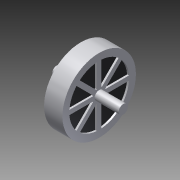
# Autodesk Inventor part: Wheel
Saved by Autodesk Inventor 2015 (Build 190159000, 159)
## iProperties
Created: 2015-01-08
Part Number: Wheel
Material: Generic
Document SubType Name: Modeling
Designer: Chandler Willoughby
Density: 1 g/cm^3
Appearance: Default
Author: Chandler Willoughby
Autodesk Inventor part; units mm, degrees
ref_plane "YZ Plane" through (0, 0, 0) normal (1, 0, 0) x (0, 1, 0)
ref_plane "XZ Plane" through (0, 0, 0) normal (0, 1, 0) x (-1, 0, 0)
ref_plane "XY Plane" through (0, 0, 0) normal (0, 0, 1) x (1, 0, 0)
sketch "Sketch1" plane through (0, 0, 0) normal (1, 0, 0) x (0, 1, 0)
  circle A0 centre (0, 0) radius 50.8
  dimension "d0" = 101.6
  constraints: 1 centre point, 1 coincident
  measures "d0" diameter of A0
extrude "Extrusion1" add sketch "Sketch1" along normal blind 25.4
sketch "Sketch2" plane through (25.4, 0, 0) normal (1, 0, 0) x (0, 0, -1)
  circle A0 centre (0, 0) radius 6.35
  dimension "d4" = 12.7
  constraints: 1 centre point, 1 coincident
  measures "d4" diameter of A0
extrude "Extrusion2" add sketch "Sketch2" along normal blind 33.3375
sketch "Sketch3" plane through (0, 0, 0) normal (-1, 0, 0) x (0, 0, 1)
  circle A0 centre (0, 0) radius 6.35
  constraints: 1 centre point, 1 coincident
extrude "Extrusion3" add sketch "Sketch3" along normal blind 33.3375
sketch "Sketch5" plane through (25.4, 0, 0) normal (1, 0, 0) x (0, 0, -1)
  circle A0 centre (0, 0) radius 44.45
  arc A1 (31.3429, -26.8561) -> (41.1529, -3.1727) centre (0, 0) ccw
  line L0 (0, 0) -> (82.55, 0) construction
  line L1 (41.1529, -3.1727) -> (8.9811, -3.1727)
  line L2 (31.3429, -26.8561) -> (82.1429, -26.8561) construction
  line L3 (31.3429, -26.8561) -> (8.594, -4.1072)
  line L4 (-4.1072, 8.594) -> (-4.5781, 9.0649)
  arc A2 (8.9811, -3.1727) -> (8.594, -4.1072) centre (8.9811, -3.7201) ccw
  arc A3 (41.1529, 3.1727) -> (31.3429, 26.8561) centre (0, 0) ccw
  line L5 (31.3429, 26.8561) -> (8.594, 4.1072)
  line L6 (41.1529, 3.1727) -> (8.9811, 3.1727)
  arc A4 (8.594, 4.1072) -> (8.9811, 3.1727) centre (8.9811, 3.7201) ccw
  arc A5 (26.8561, 31.3429) -> (3.1727, 41.1529) centre (0, 0) ccw
  line L7 (3.1727, 41.1529) -> (3.1727, 8.9811)
  line L8 (26.8561, 31.3429) -> (4.1072, 8.594)
  arc A6 (3.1727, 8.9811) -> (4.1072, 8.594) centre (3.7201, 8.9811) ccw
  arc A7 (-3.1727, 41.1529) -> (-26.8561, 31.3429) centre (0, 0) ccw
  line L9 (-26.8561, 31.3429) -> (-4.1072, 8.594)
  line L10 (-3.1727, 41.1529) -> (-3.1727, 8.9811)
  arc A8 (-4.1072, 8.594) -> (-3.1727, 8.9811) centre (-3.7201, 8.9811) ccw
  arc A9 (-31.3429, 26.8561) -> (-41.1529, 3.1727) centre (0, 0) ccw
  line L11 (-41.1529, 3.1727) -> (-8.9811, 3.1727)
  line L12 (-31.3429, 26.8561) -> (-8.594, 4.1072)
  arc A10 (-8.9811, 3.1727) -> (-8.594, 4.1072) centre (-8.9811, 3.7201) ccw
  arc A11 (-41.1529, -3.1727) -> (-31.3429, -26.8561) centre (0, 0) ccw
  line L13 (-31.3429, -26.8561) -> (-8.594, -4.1072)
  line L14 (-41.1529, -3.1727) -> (-8.9811, -3.1727)
  arc A12 (-8.594, -4.1072) -> (-8.9811, -3.1727) centre (-8.9811, -3.7201) ccw
  arc A13 (-26.8561, -31.3429) -> (-3.1727, -41.1529) centre (0, 0) ccw
  line L15 (-3.1727, -41.1529) -> (-3.1727, -8.9811)
  line L16 (-26.8561, -31.3429) -> (-4.1072, -8.594)
  arc A14 (-3.1727, -8.9811) -> (-4.1072, -8.594) centre (-3.7201, -8.9811) ccw
  arc A15 (3.1727, -41.1529) -> (26.8561, -31.3429) centre (0, 0) ccw
  line L17 (26.8561, -31.3429) -> (4.1072, -8.594)
  line L18 (3.1727, -41.1529) -> (3.1727, -8.9811)
  arc A16 (4.1072, -8.594) -> (3.1727, -8.9811) centre (3.7201, -8.9811) ccw
  dimension "d12" = 88.9
  dimension "d13" = 82.55
  dimension "d24" = 360
  constraints: 38 end point, 32 point on circle, 18 coincident, 17 centre point, 3 horizontal, 1 tangent, 95 other
  measures "d12" diameter of A0
  measures "d13" diameter of A1
extrude "Extrusion5" cut sketch "Sketch5" against normal blind 2.54 contours L3 A2 L1 A1 | L4 L9 A7 L10 A8 | L6 A4 L5 A3 | L8 A6 L7 A5 | L12 A10 L11 A9 | L14 A12 L13 A11 | L16 A14 L15 A13 | L18 A16 L17 A15
sketch "Sketch6" plane through (0, 0, 0) normal (-1, 0, 0) x (0, 0, 1)
  circle A0 centre (0, 0) radius 44.45
  arc A1 (-31.3429, 26.8561) -> (-41.1529, 3.1727) centre (0, 0) ccw
  line L0 (-8.594, 4.1072) -> (-31.3429, 26.8561) projected
  line L1 (-41.1529, 3.1727) -> (-8.9811, 3.1727)
  line L2 (-41.1529, 3.1727) -> (-8.9811, 3.1727) projected
  line L3 (-8.594, 4.1072) -> (-31.3429, 26.8561)
  arc A2 (-8.9811, 3.1727) -> (-8.594, 4.1072) centre (-8.9811, 3.7201) ccw
  arc A3 (-41.1529, -3.1727) -> (-31.3429, -26.8561) centre (0, 0) ccw
  line L4 (-31.3429, -26.8561) -> (-8.594, -4.1072)
  line L5 (-8.9811, -3.1727) -> (-41.1529, -3.1727)
  arc A4 (-8.594, -4.1072) -> (-8.9811, -3.1727) centre (-8.9811, -3.7201) ccw
  arc A5 (-26.8561, -31.3429) -> (-3.1727, -41.1529) centre (0, 0) ccw
  line L6 (-3.1727, -41.1529) -> (-3.1727, -8.9811)
  line L7 (-4.1072, -8.594) -> (-26.8561, -31.3429)
  arc A6 (-3.1727, -8.9811) -> (-4.1072, -8.594) centre (-3.7201, -8.9811) ccw
  arc A7 (3.1727, -41.1529) -> (26.8561, -31.3429) centre (0, 0) ccw
  line L8 (26.8561, -31.3429) -> (4.1072, -8.594)
  line L9 (3.1727, -8.9811) -> (3.1727, -41.1529)
  arc A8 (4.1072, -8.594) -> (3.1727, -8.9811) centre (3.7201, -8.9811) ccw
  arc A9 (31.3429, -26.8561) -> (41.1529, -3.1727) centre (0, 0) ccw
  line L10 (41.1529, -3.1727) -> (8.9811, -3.1727)
  line L11 (8.594, -4.1072) -> (31.3429, -26.8561)
  arc A10 (8.9811, -3.1727) -> (8.594, -4.1072) centre (8.9811, -3.7201) ccw
  arc A11 (41.1529, 3.1727) -> (31.3429, 26.8561) centre (0, 0) ccw
  line L12 (31.3429, 26.8561) -> (8.594, 4.1072)
  line L13 (8.9811, 3.1727) -> (41.1529, 3.1727)
  arc A12 (8.594, 4.1072) -> (8.9811, 3.1727) centre (8.9811, 3.7201) ccw
  arc A13 (26.8561, 31.3429) -> (3.1727, 41.1529) centre (0, 0) ccw
  line L14 (3.1727, 41.1529) -> (3.1727, 8.9811)
  line L15 (4.1072, 8.594) -> (26.8561, 31.3429)
  arc A14 (3.1727, 8.9811) -> (4.1072, 8.594) centre (3.7201, 8.9811) ccw
  arc A15 (-3.1727, 41.1529) -> (-26.8561, 31.3429) centre (0, 0) ccw
  line L16 (-26.8561, 31.3429) -> (-4.1072, 8.594)
  line L17 (-3.1727, 8.9811) -> (-3.1727, 41.1529)
  arc A16 (-4.1072, 8.594) -> (-3.1727, 8.9811) centre (-3.7201, 8.9811) ccw
  dimension "d28" = 88.9
  dimension "d32" = 360
  constraints: 33 end point, 32 point on circle, 17 centre point, 2 coincident, 2 collinear, 1 tangent, 81 other
  measures "d28" diameter of A0
extrude "Extrusion6" cut sketch "Sketch6" against normal blind 2.54 contours L0 A2 L1 A1 | L5 A4 L4 A3 | L7 A6 L6 A5 | L9 A8 L8 A7 | L11 A10 L10 A9 | L13 A12 L12 A11 | L15 A14 L14 A13 | L17 A16 L16 A15
body "Solid1"
